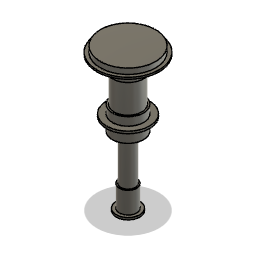
1.5W 4K v2 (Autodesk Fusion 360 design; units mm, degrees)
Autodesk Fusion 360 part; units mm, degrees
sketch "Sketch1" plane through (0, 0, 0) normal (0, 0, 1) x (1, 0, 0)
  line L0 (0, 0) -> (-34, 0)
  line L1 (-34, 0) -> (-34, 6)
  line L2 (-34, 6) -> (-25, 6)
  line L3 (-25, 6) -> (-25, 68)
  line L4 (-25, 68) -> (-21, 68)
  line L5 (-21, 68) -> (-21, 199.8)
  line L6 (-21, 199.8) -> (-45, 199.8)
  line L7 (-45, 199.8) -> (-45, 236.5)
  line L8 (-45, 236.5) -> (-62.5, 236.5)
  line L9 (-62.5, 236.5) -> (-62.5, 243)
  line L10 (-62.5, 243) -> (-45, 243)
  line L11 (-45, 243) -> (-45, 266.8)
  line L12 (-45, 266.8) -> (-40, 266.8)
  line L13 (-40, 266.8) -> (-40, 352.5)
  line L14 (-40, 352.5) -> (-45, 352.5)
  line L15 (-45, 352.5) -> (-45, 392.5)
  line L16 (-45, 392.5) -> (-90, 392.5)
  line L17 (-90, 392.5) -> (-90, 397.5)
  line L18 (-90, 397.5) -> (0, 397.5)
  line L19 (0, 397.5) -> (0, 0)
  line L20 (-80, 397.5) -> (-80, 413.5)
  line L21 (-80, 413.5) -> (0, 413.5)
  line L22 (0, 413.5) -> (0, 397.5)
  dimension "d1" = 34
  dimension "d2" = 25
  dimension "d3" = 6
  dimension "d5" = 90
  dimension "d6" = 5
  dimension "d7" = 45
  dimension "d8" = 62.5
  dimension "d9" = 6.5
  dimension "d10" = 68
  dimension "d11" = 236.5
  dimension "d12" = 67
  dimension "d13" = 192.7
  dimension "d14" = 5
  dimension "d15" = 40
  dimension "d16" = 4
  dimension "d17" = 392.5
  dimension "d18" = 21
  dimension "d19" = 10
  constraint coincident L0.start L19.end
  constraint horizontal L0
  constraint perpendicular L0 L1
  constraint perpendicular L1 L2
  constraint perpendicular L0 L3
  constraint perpendicular L3 L4
  constraint perpendicular L0 L5
  constraint perpendicular L5 L6
  constraint perpendicular L6 L7
  constraint perpendicular L7 L8
  constraint perpendicular L8 L9
  constraint perpendicular L9 L10
  constraint perpendicular L10 L11
  constraint perpendicular L11 L12
  constraint perpendicular L10 L13
  constraint perpendicular L13 L14
  constraint perpendicular L14 L15
  constraint perpendicular L15 L16
  constraint perpendicular L16 L17
  constraint perpendicular L17 L18
  constraint perpendicular L0 L19
  constraint collinear L11 L15
  constraint collinear L7 L11
  constraint coincident L18 L20.start
  constraint perpendicular L18 L20
  constraint perpendicular L17 L21
  constraint perpendicular L18 L22
  measures "d1" distance of L1 L19
  measures "d2" distance of L3 L19
  measures "d3" distance of L0 L2
  measures "d5" distance of L17 L19
  measures "d6" distance of L16 L18
  measures "d7" distance of L15 L19
  measures "d8" distance of L9 L19
  measures "d9" distance of L8 L10
  measures "d10" distance of L0 L4
  measures "d11" distance of L0 L8
  measures "d12" distance of L6 L12
  measures "d13" distance of L6 L16
  measures "d14" distance of L11 L13
  measures "d15" distance of L14 L16
  measures "d16" distance of L3 L5
  measures "d17" distance of L0 L16
  measures "d18" distance of L16 L21
  measures "d19" distance of L17.end L20
revolve "Revolve1" add sketch "Sketch1" angle 360 about axis through (0, 397.5, 0) along (0, -1, 0)
equation "d8 = ( 125 / 2 ) * 1 mm"
